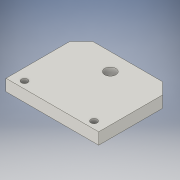
# Autodesk Inventor part: Werkstück_B
Saved by Autodesk Inventor 2018.3 (Build 223284000, 284)
## iProperties
RuleStatus: InUse
Created: 2019-11-28
Material: Stahl, unlegiert
Document SubType Name: Modeling
Designer: dirkb
Density: 7.85 g/cm^3
Appearance: Stahl
Description: Werkstück
Part Number: Werkstück_B
Werkstoff: S235JRC+C
Author: dirkb
Autodesk Inventor part; units mm, degrees
ref_plane "YZ Plane" through (0, 0, 0) normal (1, 0, 0) x (0, 1, 0)
ref_plane "XZ Plane" through (0, 0, 0) normal (0, 1, 0) x (-1, 0, 0)
ref_plane "XY Plane" through (0, 0, 0) normal (0, 0, 1) x (1, 0, 0)
sketch "Skizze_Grundkörper" plane through (0, 0, 0) normal (0, 0, 1) x (1, 0, 0)
  line L0 (-56, 0) -> (56, 0) projected
  line L1 (0, -45.5) -> (0, 45.5) projected
  line L2 (40, -32.5) -> (-40, -32.5)
  line L3 (-40, -32.5) -> (-40, 32.5)
  line L4 (-40, 32.5) -> (40, 32.5)
  line L5 (40, 32.5) -> (40, -32.5)
  line L6 (40, -32.5) -> (-40, 32.5) construction
  line L7 (-40, -32.5) -> (40, 32.5) construction
  point P0 (0, 0)
  dimension "Länge" = 80
  dimension "Höhe" = 65
  constraints: 12 end point, 2 midpoint, 2 parallel, 1 horizontal, 1 perpendicular
  measures "Länge" distance of L3.end L4.end
  measures "Höhe" distance of L4.end L2.start
extrude "Grundkörper" add sketch "Skizze_Grundkörper" along normal blind 10
sketch "Skizze2" plane through (0, 0, 10) normal (0, 0, 1) x (1, 0, 0)
  line L0 (-40, -32.5) -> (40, -32.5) projected
  line L1 (40, -32.5) -> (40, 32.5) projected
  line L2 (40, 32.5) -> (-40, 32.5) projected
  line L3 (-40, 32.5) -> (-40, -32.5) projected
  line L4 (-56, 0) -> (56, 0) projected
  line L5 (0, -45.5) -> (0, 45.5) projected
  point P0 (0, 0)
  point P1 (0, 17.5)
  dimension "d4" = 50
  constraints: 1 point on line
  measures "d4" distance from line of L0 point (0, 17.5)
hole "Bohrung_9,7_mm" at (0, 17.5, 10) direction (0, 0, -1) diameter 9.7 end through all
sketch "Skizze3" plane through (0, 0, 10) normal (0, 0, 1) x (1, 0, 0)
  circle A0 centre (0, 17.5) radius 4.85 projected
  line L0 (-40, -32.5) -> (40, -32.5) projected
  line L1 (40, -32.5) -> (40, 32.5) projected
  line L2 (40, 32.5) -> (-40, 32.5) projected
  line L3 (-40, 32.5) -> (-40, -32.5) projected
  line L4 (-56, 0) -> (56, 0) projected
  line L5 (0, -45.5) -> (0, 45.5) projected
  point P0 (0, 0)
  point P1 (-30, -26.5)
  point P2 (30, -26.5)
  dimension "d12" = 60
  dimension "d13" = 6
  constraints: 1 symmetric about line
  measures "d12" distance of point (30, -26.5) point (-30, -26.5)
  measures "d13" distance from line of L0 point (30, -26.5)
hole "Bohrung_5,5_mm" at (-30, -26.5, 10) at (30, -26.5, 10) direction (0, 0, -1) diameter 5.5 end through all
chamfer "Fase_10_mm" distance 10 angle 45 2 edges at (-40, 32.5, 5) (40, 32.5, 5)
